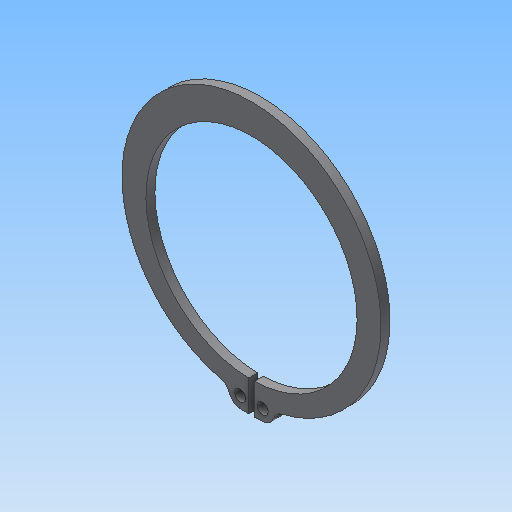
# Autodesk Inventor part: R-Ring50
Saved by Autodesk Inventor 2020.1 (Build 241239000, 239)
## iProperties
Comments: To add or edit properties for Autodesk Inventor files, use iProperties.
Shininess: 64.0
Length Units: 11269
Angle Units: 11279
Time Units: 11290
Mass Units: 11283
Length Display Precision: 3
Angle Display Precision: 2
Compacted: True
Alert: To add or edit properties for Autodesk Inventor files, use iProperties.
Component Type: 1
Library Location: C:\Programme\Autodesk\Inventor 6\content
Library: local
SubLibrary: DIN
Family: 299
Member: 540
Member Major Revision: 1
Member Minor Revision: 2
Created: 2003-03-06
Part Number: R-Ring50
Vendor: Autodesk Inc.
Document SubType Name: Modeling
Designer: rueghs
Description: Sicherungsring
Standard: DIN 471 50 x 2
Material: Generic
Density: 1 g/cm^3
Appearance: Default
Density: 0.0
Volumn: 0.0
Area: 0.0
PropertySet Name: Model Information
Control State: 0
Master: False
Checked Out: False
Author: rueghs
Revision Number: 2
Autodesk Inventor part; units mm, degrees
ref_plane "YZ Plane" through (0, 0, 0) normal (1, 0, 0) x (0, 1, 0)
ref_plane "XZ Plane" through (0, 0, 0) normal (0, 1, 0) x (-1, 0, 0)
ref_plane "XY Plane" through (0, 0, 0) normal (0, 0, 1) x (1, 0, 0)
sketch "Skizze1" plane through (0, 0, 0) normal (0, 0, 1) x (1, 0, 0)
  line L0 (-6, 0) -> (6, 0) construction
  arc A0 (0.625, -48.4917) -> (-0.625, -48.4917) centre (0, -25) ccw
  line L1 (0, 23.3134) -> (0, -61.6825) projected
  line L2 (-34.59, 0) -> (46.12, 0) projected
  line L3 (-0.625, -48.4917) -> (-0.625, -55.3917)
  line L4 (-0.625, -6.5402) -> (-0.625, -13.29) construction
  line L5 (-2.7947, 5.1) -> (3.6722, 5.1) construction
  arc A1 (6.7169, -51.7565) -> (-6.7169, -51.7565) centre (0, -23.725) ccw
  arc A2 (-2.724, -55.2758) -> (-0.625, -55.3917) centre (0, -25) ccw
  arc A3 (-4.8997, -53.4868) -> (-2.724, -55.2758) centre (-2.5, -52.7859) ccw
  arc A4 (-4.8997, -53.4868) -> (-6.7169, -51.7565) centre (-7.2995, -54.1877) ccw
  line L6 (0.625, -48.4917) -> (0.625, -55.3917)
  line L7 (0.625, -6.5402) -> (0.625, -13.29) construction
  arc A5 (0.625, -55.3917) -> (2.724, -55.2758) centre (0, -25) ccw
  arc A6 (2.724, -55.2758) -> (4.8997, -53.4868) centre (2.5, -52.7859) ccw
  arc A7 (6.7169, -51.7565) -> (4.8997, -53.4868) centre (7.2995, -54.1877) ccw
  circle A8 centre (-2.5, -52.7859) radius 1.25
  circle A9 centre (2.5, -52.7859) radius 1.25
  dimension "d0" = 47
  dimension "d1" = 6.9
  dimension "d6" = 0.625
  dimension "d7" = 5.1
  dimension "d8" = 1.275
  dimension "d9" = 2.5
  dimension "d10" = 2.5
  dimension "d11" = 1.875
  dimension "d12" = 2.5
  dimension "d13" = 2.5
  dimension "d14" = 25
  constraints: 16 point on circle, 12 end point, 10 centre point, 9 symmetric about line, 5 point on line, 4 tangent, 3 coincident, 2 horizontal, 1 perpendicular, 1 vertical, 5 other
  measures "d0" diameter of A0
  measures "d1" distance of L3.end L3.start
  measures "d6" distance between parallel lines of L1 L4
  measures "d7" distance between parallel lines of L5 L2
  measures "d8" distance of A0.centre A1.centre
  measures "d9" radius of A3
  measures "d10" radius of A4
  measures "d11" distance from line of L3 A3.centre
  measures "d12" diameter of A8
  measures "d13" diameter of A9
  measures "d14" distance from line of A0.centre L0
extrude "Körper" add sketch "Skizze1" along normal blind 2
equation "\"d0\" = ND"
equation "\"d1\" = SRB2"
equation "\"d6\" = 0.25 * SD5"
equation "\"d7\" = SRB1"
equation "\"d8\" = 0.25 * SRB1"
equation "\"d9\" = SD5"
equation "\"d10\" = SD5"
equation "\"d11\" = 0.75 * SD5"
equation "\"d12\" = SD5"
equation "\"d13\" = SD5"
equation "\"d14\" = 0.5 * WD"
equation "\"d2\" = SD"
equation "\"SD\" = 2"
equation "\"SRB1\" = 5.1"
equation "\"ND\" = 47"
equation "\"SRB2\" = 6.9"
equation "\"SD5\" = 2.5"
equation "\"SD3\" = 45.8"
equation "\"WDMAX\" = 52"
equation "\"WD\" = 50"
body "Solid1"
